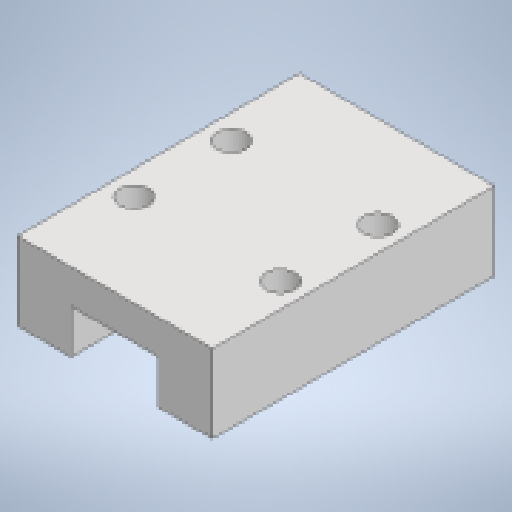
# Autodesk Inventor part: MGN9C_block
Saved by Autodesk Inventor 2024 (Build 280153000, 153)
## iProperties
Created: 2023-08-11
Part Number: MGN9C_block
Material: Generic
Document SubType Name: Modeling
Designer: l1534
Density: 1 g/cm^3
Appearance: Default
Author: l1534
Autodesk Inventor part; units mm, degrees
ref_plane "YZ Plane" through (0, 0, 0) normal (1, 0, 0) x (0, 1, 0)
ref_plane "XZ Plane" through (0, 0, 0) normal (0, 1, 0) x (-1, 0, 0)
ref_plane "XY Plane" through (0, 0, 0) normal (0, 0, 1) x (1, 0, 0)
sketch "Sketch1" plane through (0, 0, 0) normal (0, 0, 1) x (1, 0, 0)
  line L0 (-9.7813, 0.4833) -> (-4.2813, 0.4833)
  line L1 (-4.2813, 0.4833) -> (-4.2813, 4.9833)
  line L2 (-4.2813, 4.9833) -> (4.7187, 4.9833)
  line L3 (4.7187, 4.9833) -> (4.7187, 0.4833)
  line L4 (4.7187, 0.4833) -> (10.2187, 0.4833)
  line L5 (10.2187, 0.4833) -> (10.2187, 8.4833)
  line L6 (10.2187, 8.4833) -> (-9.7813, 8.4833)
  line L7 (-9.7813, 8.4833) -> (-9.7813, 0.4833)
  point P0 (0, 0)
  dimension "d0" = 20
  dimension "d1" = 8
  dimension "d2" = 4.5
  dimension "d3" = 9
  dimension "d4" = 5.5
  constraints: 16 end point, 5 perpendicular, 2 point on line, 1 horizontal, 1 parallel
  measures "d0" distance of L5.end L6.end
  measures "d1" distance of L4.end L5.end
  measures "d2" distance of L2.end L3.end
  measures "d3" distance of L1.end L2.end
  measures "d4" distance of L3.end L4.end
extrude "Extrusion1" add sketch "Sketch1" along normal blind 28.9
sketch "Sketch2" plane through (-9.7813, 8.4833, 0) normal (0, 1, 0) x (1, 0, 0)
  circle A0 centre (2.5, -9.45) radius 1.5
  circle A1 centre (17.5, -9.45) radius 1.5
  circle A2 centre (17.5, -19.45) radius 1.5
  circle A3 centre (2.5, -19.45) radius 1.5
  line L0 (20, 0) -> (0, 0) projected
  line L1 (0, 0) -> (0, -28.9) projected
  line L2 (20, 0) -> (20, -28.9) projected
  point P0 (9.7813, 0)
  dimension "d7" = 3
  dimension "d8" = 3
  dimension "d9" = 3
  dimension "d10" = 3
  dimension "d11" = 9.45
  dimension "d12" = 9.45
  dimension "d13" = 10
  dimension "d14" = 10
  dimension "d15" = 2.5
  dimension "d16" = 2.5
  dimension "d18" = 2.5
  dimension "d19" = 2.5
  constraints: 4 centre point
  measures "d7" diameter of A0
  measures "d8" diameter of A1
  measures "d9" diameter of A3
  measures "d10" diameter of A2
  measures "d11" distance from line of L0 A0.centre
  measures "d12" distance from line of L0 A1.centre
  measures "d13" distance of A3.centre A0.centre
  measures "d14" distance of A1.centre A2.centre
  measures "d15" distance from line of L1 A0.centre
  measures "d16" distance from line of L1 A3.centre
  measures "d18" distance from line of L2 A1.centre
  measures "d19" distance from line of L2 A2.centre
extrude "Extrusion2" cut sketch "Sketch2" against normal blind 8
body "Solid1"
